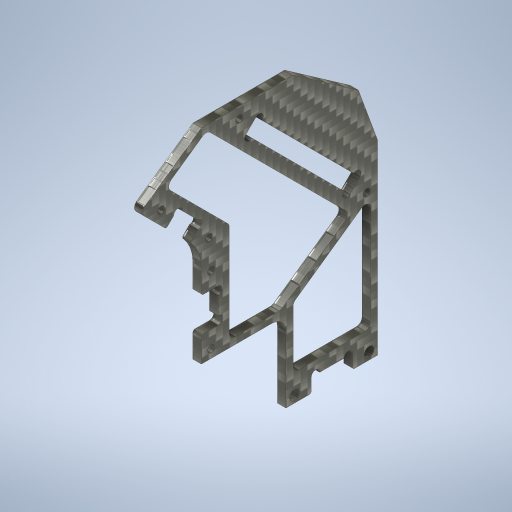
# Autodesk Inventor part: HeadSideFrame
Saved by Autodesk Inventor 2024.2 (Build 282272000, 272)
## iProperties
Created: 2024-01-28
Part Number: HeadSideFrame
Material: CFRP
Document SubType Name: Modeling
Designer: Masato Kubotera
Density: 1.43 g/cm^3
Appearance: Carbon Fiber 1
Mass: 10.5439 g
Surface Area: 75.0811 cm^2
Volume: 7.37334 cm^3
Vendor: meviy
Author: Masato Kubotera
Autodesk Inventor part; units mm, degrees
ref_plane "YZ Plane" through (0, 0, 0) normal (1, 0, 0) x (0, 1, 0)
ref_plane "XY Plane" through (0, 0, 0) normal (0, 0, 1) x (1, 0, 0)
ref_plane "Work Plane1" through (0, 30, 0) normal (0, 1, 0) x (-1, 0, 0)
sketch "Sketch1" plane through (0, 30, 0) normal (0, 1, 0) x (-1, 0, 0)
  line L0 (-16.25, -1.5) -> (16.25, -1.5)
  line L1 (-7.3, -1.5) -> (-7.3, 3.5)
  line L2 (7.3, 3.5) -> (7.3, -1.5)
  arc A0 (7.3, 3.5) -> (4.3, 3.5) centre (5.8, 3.5) ccw
  arc A1 (-4.3, 3.5) -> (-7.3, 3.5) centre (-5.8, 3.5) ccw
  line L3 (0, -1.5) -> (0, 3.5) construction
  line L4 (-13.25, 1) -> (13.25, 1) construction
  line L5 (-7.25, -1.5) -> (-7.25, 3.5) construction
  line L6 (7.25, -1.5) -> (7.25, 3.5) construction
  arc A2 (-47.5142, 68.9298) -> (-47.5142, 71.9298) centre (-47.5142, 70.4298) ccw
  line L7 (-62.6665, 83.5467) -> (-41.4533, 62.3335) construction
  line L8 (-33.1802, 70.6066) -> (-54.3934, 91.8198) construction
  line L9 (-53.8277, 71.1723) -> (-50.2922, 74.7078) construction
  arc A3 (-53.0702, 77.4858) -> (-56.0702, 77.4858) centre (-54.5702, 77.4858) ccw
  line L10 (-49.5851, 66.9296) -> (-46.0495, 70.4652) construction
  line L11 (-54.5348, 78.9505) -> (-49.5851, 66.9296) construction
  line L12 (-46.0495, 70.4652) -> (-54.5348, 78.9505) construction
  line L13 (-46.0495, 70.4652) -> (-58.0704, 75.4149) construction
  line L14 (-54.5348, 78.9505) -> (-58.0704, 75.4149) construction
  line L15 (-58.0704, 75.4149) -> (-49.5851, 66.9296) construction
  line L16 (-54.5702, 78.9858) -> (-58.7421, 74.8139)
  line L17 (-62.7373, 50.2419) -> (-46.0495, 66.9296) construction
  line L18 (-41.4533, 62.3335) -> (-33.1802, 70.6066) construction
  line L19 (-46.0142, 70.4298) -> (-54.5702, 78.9858)
  line L20 (-60.5452, 81.4253) -> (-43.5747, 64.4548) construction
  line L21 (-74.7581, 62.2627) -> (-62.7373, 50.2419) construction
  line L22 (-58.0704, 78.9505) -> (-74.7581, 62.2627) construction
  line L23 (-54.3934, 91.8198) -> (-62.6665, 83.5467) construction
  line L24 (-65, 60) -> (-125, 0) construction
  line L25 (0, 0) -> (-125, 0) construction
  line L26 (10.1236, 102) -> (65.1439, 102) construction
  line L27 (-7.3, 3.5) -> (7.3, 3.5)
  line L28 (-46.25, 102) -> (-46.25, 27) construction
  ellipse E0 centre (-46.25, 64.5) end of major axis (-46.25, 102) minor radius 30 (-46.25, 102) -> (-46.25, 27) ccw construction
  line L29 (-30, 102) -> (-30, 27) construction
  ellipse E1 centre (-13.75, 64.5) end of major axis (-13.75, 102) minor radius 30 (-13.75, 27) -> (-13.75, 102) ccw construction
  line L30 (-46.25, 102) -> (-13.75, 102) construction
  line L31 (-46.25, 27) -> (-13.75, 27) construction
  line L32 (-58.9896, 53.9896) -> (-71.0104, 66.0104) construction
  line L33 (-57.5883, 37.2154) -> (-87.7846, 67.4117) construction
  line L34 (-65, 60) -> (-57.5883, 37.2154) construction
  line L35 (-65, 60) -> (-87.7846, 67.4117) construction
  line L36 (-46.0142, 70.4298) -> (-50.1861, 66.2579)
  line L37 (-58.7421, 74.8139) -> (-68.1169, 84.1887)
  line L38 (16.25, -1.5) -> (16.25, 64.5)
  line L39 (-16.25, -1.5) -> (-16.25, 27)
  line L40 (-30.419, 89.6005) -> (-26.8835, 93.136) construction
  line L41 (-26.8835, 93.136) -> (9.886, 56.3665) construction
  line L42 (9.886, 56.3665) -> (6.3505, 52.831) construction
  line L43 (6.3505, 52.831) -> (-30.419, 89.6005) construction
  line L44 (-30.419, 89.6005) -> (9.886, 56.3665) construction
  line L45 (-26.8835, 93.136) -> (6.3505, 52.831) construction
  line L46 (-30.4898, 89.6005) -> (-26.8835, 93.2067)
  line L47 (-26.8835, 93.2067) -> (9.9567, 56.3665)
  line L48 (9.9567, 56.3665) -> (6.3505, 52.7602)
  line L49 (6.3505, 52.7602) -> (-30.4898, 89.6005)
  line L50 (-30.4898, 89.6005) -> (9.9567, 56.3665) construction
  line L51 (-26.8835, 93.2067) -> (6.3505, 52.7602) construction
  arc A4 (-24.7622, 91.0854) -> (-26.8835, 93.2067) centre (-25.8229, 92.1461) ccw
  line L52 (-35.0152, 97.7322) -> (14.4822, 48.2348) construction
  line L53 (-8.4634, 74.7866) -> (-12.0696, 71.1804) construction
  arc A5 (-30.4898, 89.6005) -> (-28.3684, 87.4792) centre (-29.4291, 88.5398) ccw
  arc A6 (9.9567, 56.3665) -> (7.8354, 58.4878) centre (8.8961, 57.4271) ccw
  arc A7 (4.2292, 54.8816) -> (6.3505, 52.7602) centre (5.2898, 53.8209) ccw
  line L54 (-46.25, 56.7553) -> (-46.25, 27)
  line L55 (-33.2475, 99.5) -> (-36.783, 95.9645) construction
  line L56 (-40.35, 36) -> (-46.25, 36) construction
  line L57 (-46.25, 48) -> (-40.35, 48) construction
  line L58 (-40.35, 48) -> (-40.35, 36) construction
  line L59 (-40.35, 36) -> (-46.25, 48) construction
  line L60 (-46.25, 36) -> (-40.35, 48) construction
  line L61 (-46.25, 48.05) -> (-40.35, 48.05)
  line L62 (-40.35, 48.05) -> (-40.35, 35.95)
  line L63 (-40.35, 35.95) -> (-46.25, 35.95)
  line L64 (-40.35, 42) -> (-46.25, 42) construction
  arc A8 (-40.35, 45.05) -> (-40.35, 48.05) centre (-40.35, 46.55) ccw
  line L65 (-42.85, 54) -> (-42.85, 30) construction
  line L66 (-46.25, 57) -> (-40.35, 57) construction
  arc A9 (-40.35, 35.95) -> (-40.35, 38.95) centre (-40.35, 37.45) ccw
  line L67 (-65.0707, 81.1425) -> (-60.8988, 85.3144) construction
  line L68 (-43.2211, 60.5657) -> (-39.6856, 64.1012) construction
  line L69 (-46.25, 64.5) -> (-76.25, 64.5) construction
  line L70 (-13.75, 64.5) -> (16.25, 64.5) construction
  line L71 (-11.75, 8) -> (11.75, 8)
  line L72 (-46.25, 99.5) -> (-13.75, 99.5)
  line L73 (-50.1861, 66.2579) -> (-46.25, 70.194)
  circle A10 centre (-42.85, 30) radius 2.4 construction
  circle A11 centre (-60.5452, 81.4253) radius 2.4 construction
  line L74 (-50.1861, 66.2579) -> (-50.1861, 66.2579)
  line L75 (-36.35, 64.0941) -> (-36.35, 31.5)
  line L76 (4.9456, 48.5083) -> (-43.1484, 96.6023)
  line L77 (-36.9358, 65.5083) -> (-57.284, 85.8565)
  line L78 (-18.7392, 29.5) -> (-34.35, 29.5)
  line L79 (9.4147, 83.2799) -> (16.25, 64.5)
  line L80 (-13.75, 102) -> (-13.75, 27) construction
  line L81 (-13.75, 99.5) -> (9.4147, 83.2799)
  line L82 (16.25, 64.5) -> (9.4147, 45.7201)
  line L83 (9.4147, 45.7201) -> (-12.8972, 30.0972)
  line L84 (-46.25, 27) -> (-16.25, 27)
  line L85 (-13.75, 28.4589) -> (-13.75, 10)
  line L86 (13.75, 10) -> (13.75, 44.9137)
  line L87 (-46.25, 99.5) -> (-68.1169, 84.1887)
  line L88 (9.4147, 45.7201) -> (10.6028, 46.552)
  line L89 (4.6786, 45.4558) -> (-17.5921, 29.8617)
  line L90 (-57.0169, 88.909) -> (-45.7097, 96.8264)
  arc A12 (-43.1484, 96.6023) -> (-45.7097, 96.8264) centre (-44.5626, 95.1881) ccw
  arc A13 (-57.0169, 88.909) -> (-57.284, 85.8565) centre (-55.8698, 87.2707) ccw
  arc A14 (4.6786, 45.4558) -> (4.9456, 48.5083) centre (3.5314, 47.0941) ccw
  arc A15 (-18.7392, 29.5) -> (-17.5921, 29.8617) centre (-18.7392, 31.5) ccw
  arc A16 (-36.35, 31.5) -> (-34.35, 29.5) centre (-34.35, 31.5) ccw
  arc A17 (13.75, 44.9137) -> (10.6028, 46.552) centre (11.75, 44.9137) ccw
  arc A18 (-12.8972, 30.0972) -> (-13.75, 28.4589) centre (-11.75, 28.4589) ccw
  arc A19 (-13.75, 10) -> (-11.75, 8) centre (-11.75, 10) ccw
  arc A20 (11.75, 8) -> (13.75, 10) centre (11.75, 10) ccw
  arc A21 (-46.25, 56.7553) -> (-50.1861, 66.2579) centre (-59.6887, 56.7553) ccw
  line L91 (12.7145, 46.467) -> (16.25, 50.0025) construction
  arc A22 (-36.35, 64.0941) -> (-36.9358, 65.5083) centre (-38.35, 64.0941) ccw
  point P0 (-52.0599, 72.9401)
  point P1 (-47.5142, 71.9298)
  point P2 (-72.6865, 52.3135)
  point P3 (-76.2424, 63.6571)
  point P4 (-75.2442, 54.8713)
  point P5 (-46.0142, 70.4298)
  point P6 (-47.5142, 68.9298)
  point P7 (-46.0142, 70.4298)
  point P8 (-16.25, 34)
  point P9 (-10.2665, 72.9835)
  point P10 (-46.25, 62.3218)
  point P11 (-32.8939, 95.6109)
  point P12 (12.3609, 50.3561)
  point P13 (7.8354, 58.4878)
  point P14 (4.2292, 54.8816)
  point P15 (-28.3684, 87.4792)
  point P16 (-43.3, 42)
  point P17 (-40.35, 34.95)
  point P18 (-73.75, 64.5)
  point P19 (-13.75, 8)
  point P20 (13.75, 8)
  point P21 (16.25, 71.5)
  point P22 (-40.35, 38.95)
  point P23 (-47.0041, 71.6114)
  point P24 (6.631, 46.8229)
  point P25 (-36.35, 67.4368)
  point P26 (-36.35, 29.5)
  point P27 (-44.335, 97.7889)
  point P28 (-71.25, 64.5)
  point P29 (-39.3749, 67.9474)
  point P30 (-58.9694, 87.5419)
  point P31 (-13.75, 29.5)
  point P32 (13.75, 57.6313)
  point P33 (13.75, 48.7557)
  point P34 (-18.1086, 29.5)
  point P35 (-36.35, 64.9225)
  point P36 (-50.1861, 66.2579)
  dimension "d26" = 30
  dimension "d1" = 32.5
  dimension "d2" = 1.5
  dimension "d3" = 1.5
  dimension "d4" = 0.05
  dimension "d5" = 6
  dimension "d6" = 11.7
  dimension "d7" = 35.3
  dimension "d8" = 30
  dimension "d9" = 17
  dimension "d10" = 30
  dimension "d11" = 0.05
  dimension "d12" = 5
  dimension "d14" = 6
  dimension "d15" = 45
  dimension "d16" = 65
  dimension "d17" = 60
  dimension "d18" = 102
  dimension "d19" = 1.5
  dimension "d20" = 2.5
  dimension "d22" = 5
  dimension "d24" = 75
  dimension "d25" = 30
  dimension "d32" = 84.8528
  dimension "d34" = 10.8703
  dimension "d35" = 21.352
  dimension "d44" = 32.5
  dimension "d50" = 9
  dimension "d55" = 5
  dimension "d56" = 52
  dimension "d60" = 6
  dimension "d61" = 0.05
  dimension "d62" = 0.05
  dimension "d64" = 0.05
  dimension "d67" = 5.9
  dimension "d68" = 6
  dimension "d70" = 9
  dimension "d71" = 9
  dimension "d75" = 2.5
  dimension "d76" = 30
  dimension "d81" = 3
  dimension "d96" = 4.8
  dimension "d97" = 0.6
  dimension "d98" = 15
  dimension "d99" = 2.5
  dimension "d100" = 1
  dimension "d101" = 1
  dimension "d103" = 2.5
  dimension "d106" = 2.5
  dimension "d109" = 145
  dimension "d110" = 145
  dimension "d111" = 2.5
  dimension "d112" = 140
  dimension "d113" = 2
  dimension "d117" = 2.5
  dimension "d118" = 2.5
  dimension "d119" = 2.5
  dimension "d120" = 70
  dimension "d121" = 45
  dimension "d122" = 30
  dimension "d123" = 4
  constraints: 186 end point, 71 point on line, 43 point on circle, 24 midpoint, 23 centre point, 23 symmetric about line, 22 tangent, 16 parallel, 14 horizontal, 14 perpendicular, 9 coincident, 9 collinear, 8 equal radius, 8 vertical, 27 other
  measures "d1" distance of L0.start L0.end
  measures "d2" radius of A0
  measures "d3" distance from line of L0 L25.start
  measures "d4" distance between parallel lines of L2 L6
  measures "d5" distance from line of point (13.25, 1) L6
  measures "d6" distance of L7.end L8.start
  measures "d7" distance between parallel lines of L21 L8
  measures "d8" distance from line of L34.start L8
  measures "d9" distance between parallel lines of L17 L22
  measures "d10" distance of L8.start L8.end
  measures "d11" distance between parallel lines of L16 L14
  measures "d12" distance between parallel lines of L15 L12
  measures "d14" distance from line of L20.start L14
  measures "d15" angle of L24 L3
  measures "d16" horizontal distance of L25.start L34.start
  measures "d17" vertical distance of L25.start L34.start
  measures "d18" distance from line of L25.start L26
  measures "d19" radius of A3
  measures "d20" distance between parallel lines of L12 L7
  measures "d22" distance between parallel lines of L0 L27
  measures "d24" distance of L28.start L31.start
  measures "d25" distance from line of L25.start L29
  measures "d32" distance of L34.start L25.end
  measures "d34" distance from line of L33 L34.start
  measures "d35" distance of point (-72.686, 52.314) L33.end
  measures "d44" distance of L31.start L31.end
  measures "d50" distance from line of L0.end L6
  measures "d55" distance of L40.start L40.end
  measures "d56" distance of L40.end L41.end
  measures "d60" distance from line of L40 point (-32.894, 95.611)
  measures "d61" distance between parallel lines of L46 L40
  measures "d62" distance between parallel lines of L41 L47
  measures "d64" distance between parallel lines of L57 L61
  measures "d67" distance of L61.start L61.end
  measures "d68" distance from line of L57 L65.start
  measures "d70" distance between parallel lines of L57 L66
  measures "d71" distance between parallel lines of L67 L14
  measures "d75" distance of L69.end point (-73.75, 64.5)
  measures "d76" diameter of L66 L64
  measures "d81" distance edge to line of A0 L71
  measures "d96" diameter of A10
  measures "d97" distance edge to line of A10 L31
  measures "d98" distance between parallel lines of L31 L64
  measures "d99" distance between parallel lines of L62 L65
  measures "d100" distance edge to line of A10 L54
  measures "d101" distance edge to line of A11 L37
  measures "d103" distance edge to line of A9 L75
  measures "d106" distance of point (-73.75, 64.5) point (-71.25, 64.5)
  measures "d109" angle of L79 L81
  measures "d110" angle of L81 L72
  measures "d111" distance between parallel lines of L72 L30
  measures "d112" angle of L82 L79
  measures "d113" radius of A12
  measures "d117" distance between parallel lines of L83 L89
  measures "d118" distance between parallel lines of L87 L90
  measures "d119" distance edge to line of A2 L77
  measures "d120" distance between parallel lines of L91 L55
  measures "d121" angle of L29 L52
  measures "d122" distance between parallel lines of L68 L67
  measures "d123" distance between parallel lines of L76 L49
extrude "Extrusion1" add sketch "Sketch1" against normal blind 3 contours L39 L84 L54 L63 A9 L62 A8 L61 A21 L36 A2 L19 A3 L16 L37 L87 L72 L81 L79 L38 L0 L2 A0 L27 A1 L1
hole "Phi3.5" at (13.25, 30, 1) at (-13.25, 30, 1) direction (0, -1, 0) diameter 3.5 end through all
hole "Phi2.5" at (60.5452, 30, 81.4253) at (43.5747, 30, 64.4548) at (65, 30, 60) at (32.8939, 30, 95.6109) at (-12.3609, 30, 50.3561) at (42.85, 30, 54) at (42.85, 30, 30) at (73.75, 30, 64.5) direction (0, -1, 0) diameter 2.5 end through all
fillet "R5" radius 5 1 edges at (16.25, 28.5, 27)
fillet "R2" radius 2 1 edges at (68.1169, 28.5, 84.1887)
chamfer "C0.5" distance 0.5 angle 45 6 edges at (58.7421, 28.5, 74.8139) (46.25, 28.5, 35.95) (46.25, 28.5, 48.05) (7.3, 28.5, -1.5) (-7.3, 28.5, -1.5) (50.1861, 28.5, 66.2579)
equation "\"d11\" = d28"
equation "\"d28\" = 0.05"
body "Solid1"
